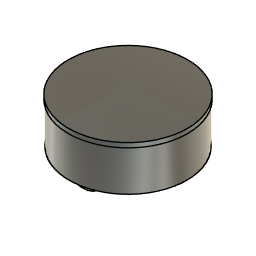
myrobot_1100404 (Autodesk Fusion 360 design; units mm, degrees)
Autodesk Fusion 360 part; units mm, degrees
sketch "Sketch1" plane through (0, 0, 0) normal (0, 0, 1) x (1, 0, 0)
  line L0 (-80, 80) -> (80, 80)
  line L1 (80, 80) -> (80, -80)
  line L2 (80, -80) -> (-80, -80)
  line L3 (-80, -80) -> (-80, 80)
  line L4 (-80, 80) -> (80, -80) construction
  line L5 (80, 80) -> (-80, -80) construction
  constraint horizontal L0
  constraint perpendicular L0 L1
  constraint parallel L0 L2
  constraint parallel L1 L3
  constraint coincident L4 origin
  constraint coincident L5 origin
extrude "Extrude1" add sketch "Sketch1" along normal blind 70 makes body 1
sketch "Sketch2" plane through (0, 0, 70) normal (0, 0, 1) x (-1, 0, 0)
  line L0 (80, 80) -> (-80, 80)
  line L1 (-80, 80) -> (-80, -80)
  line L2 (-80, -80) -> (80, -80)
  line L3 (80, -80) -> (80, 80)
sketch "Sketch3" plane through (0, 0, 70) normal (0, 0, 1) x (-1, 0, 0)
sketch "Sketch4" plane through (0, -80, 0) normal (0, -1, 0) x (1, 0, 0)
  line L0 (-80, 0) -> (80, 0)
  line L1 (80, 0) -> (80, 70)
  line L2 (80, 70) -> (-80, 70)
  line L3 (-80, 70) -> (-80, 0)
  circle A0 centre (0, 0) radius 50
  constraint coincident A0.centre origin
extrude "Extrude2" add sketch "Sketch4" along normal blind 20 separate body contours L0 A0 | L0 A0 makes body 2
mirror "Mirror1" about plane through (0, 0, 0) normal (0, 1, 0) of bodies 2 makes body 3
sketch "Sketch5" plane through (0, 0, 70) normal (0, 0, 1) x (-1, 0, 0)
  circle A0 centre (0, 0) radius 130
  constraint coincident A0.centre origin
extrude "Extrude3" add sketch "Sketch5" against normal blind 90 thin wall 1 inside separate body makes body 4
sketch "Sketch6" plane through (0, 0, 70) normal (0, 0, 1) x (-1, 0, 0)
  circle A0 centre (0, 0) radius 131.5643
  constraint coincident A0.centre origin
extrude "Extrude4" add sketch "Sketch6" along normal blind 10 bodies 1 4
sketch "Sketch7" plane through (0, 0, 0) normal (0, 0, -1) x (1, 0, 0)
  line L0 (80, 80) -> (-80, 80)
  line L1 (-80, 80) -> (-80, -80)
  line L2 (-80, -80) -> (80, -80)
  line L3 (80, -80) -> (80, 80)
  circle A0 centre (70, 0) radius 10
  circle A1 centre (-70, 0) radius 10
  constraint tangent L1 A1
extrude "Extrude5" add sketch "Sketch7" along normal blind 50 contours A1 | A0 bodies 1
fillet "Fillet1" radius 10 2 faces at (-68.1708, -0.7179, -50) (67.0145, 3.6482, -50) on bodies 1
sketch "Sketch8" plane through (0, 0, 0) normal (0, 0, -1) x (1, 0, 0)
sketch "Sketch9" plane through (0, 0, 70) normal (0, 0, -1) x (1, 0, 0)
  line L0 (-80, -80) -> (-80, 80)
  line L1 (-80, 80) -> (80, 80)
  line L2 (80, 80) -> (80, -80)
  line L3 (80, -80) -> (-80, -80)
  circle A0 centre (0, 0) radius 129
  circle A1 centre (110, 0) radius 10
move_body "Move2" bodies 1 2 3 to x (1, 0, 0) y (0, 1, 0) z (0, 0, 1) at (0, 0, 50)
sketch "Sketch10" plane through (0, 0, 120) normal (0, 0, -1) x (1, 0, 0)
  line L0 (-80, -80) -> (-80, 80)
  line L1 (-80, 80) -> (80, 80)
  line L2 (80, 80) -> (80, -80)
  line L3 (80, -80) -> (-80, -80)
  circle A0 centre (0, 0) radius 129
  circle A1 centre (110, 0) radius 10
extrude "Extrude7" add sketch "Sketch10" along normal blind 90 contours A1 bodies 1
extrude "Extrude8" add 1 faces at (107.4279, -1.414, 30) along direction (0, 0, -1) blind 10 separate body on bodies 1 makes body 5
copy_body "Body->Comp9" bodies 1 removing the originals makes body 6 in component "base_link"
copy_body "Body->Comp10" bodies 2 removing the originals makes body 7 in component "right_wheel"
copy_body "Body->Comp11" bodies 3 removing the originals makes body 8 in component "left_wheel"
copy_body "Body->Comp12" bodies 5 removing the originals makes body 9 in component "lidar"
component "base_link" placed x (1, 0, 0) y (0, 1, 0) z (0, 0, 1) at (0, 0, 0)
component "right_wheel" placed x (1, 0, 0) y (0, 1, 0) z (0, 0, 1) at (0, 0, 0)
component "left_wheel" placed x (1, 0, 0) y (0, 1, 0) z (0, 0, 1) at (0, 0, 0)
component "lidar" placed x (1, 0, 0) y (0, 1, 0) z (0, 0, 1) at (0, 0, 0)
named bodies: "base_link", "right_wheel", "left_wheel", "lidar"
